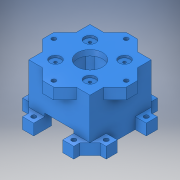
# Autodesk Inventor part: motor_holder
Saved by Autodesk Inventor 2019 (Build 230136000, 136)
## iProperties
Created: 2019-12-22
Part Number: motor_holder
Material: Пластик АБС
Document SubType Name: Modeling
Designer: Петров Иван
Density: 1.06 g/cm^3
Appearance: Голубой
Author: Петров Иван
Autodesk Inventor part; units mm, degrees
ref_plane "YZ Plane" through (0, 0, 0) normal (1, 0, 0) x (0, 1, 0)
ref_plane "XZ Plane" through (0, 0, 0) normal (0, 1, 0) x (-1, 0, 0)
ref_plane "XY Plane" through (0, 0, 0) normal (0, 0, 1) x (1, 0, 0)
sketch "Эскиз1" plane through (0, 0, 0) normal (0, 1, 0) x (-1, 0, 0)
  line L0 (-18.0075, 21.609) -> (-21.609, 18.0075)
  line L1 (-21.609, -18.0075) -> (-18.0075, -21.609)
  line L2 (18.0075, -21.609) -> (21.609, -18.0075)
  line L3 (21.609, -18.0075) -> (21.609, 18.0075)
  line L4 (21.609, 18.0075) -> (18.0075, 21.609)
  line L5 (18.0075, 21.609) -> (-18.0075, 21.609)
  circle A0 centre (0, 0) radius 11.3
  circle A1 centre (-15.5, -15.5) radius 1.25
  circle A2 centre (15.5, -15.5) radius 1.25
  circle A3 centre (15.5, 15.5) radius 1.25
  circle A4 centre (-15.5, 15.5) radius 1.25
  line L6 (13.4172, 20.8) -> (6, 20.8)
  line L7 (20.8, 13.4172) -> (13.4172, 20.8)
  line L8 (20.8, -13.4172) -> (20.8, 13.4172)
  line L9 (13.4172, -20.8) -> (20.8, -13.4172)
  line L10 (-13.4172, -20.8) -> (13.4172, -20.8)
  line L11 (-20.8, -13.4172) -> (-13.4172, -20.8)
  line L12 (-20.8, 13.4172) -> (-20.8, -13.4172)
  line L13 (-13.4172, 20.8) -> (-20.8, 13.4172)
  line L14 (-6, 20.8) -> (-13.4172, 20.8)
  line L15 (-21.609, 18.0075) -> (-21.609, -18.0075)
  line L16 (-18.0075, -21.609) -> (18.0075, -21.609)
  line L17 (-27.5, 27.5) -> (27.5, 27.5)
  line L18 (27.5, 27.5) -> (27.5, -27.5)
  line L19 (27.5, -27.5) -> (-27.5, -27.5)
  line L20 (-27.5, -27.5) -> (-27.5, 27.5)
  line L21 (-27.5, 27.5) -> (27.5, -27.5) construction
  line L22 (27.5, 27.5) -> (-27.5, -27.5) construction
  line L23 (-6, 20.8) -> (6, 20.8)
  point P0 (0, 0)
  dimension "d0" = 55
  constraints: 48 end point, 5 centre point, 2 midpoint, 2 parallel, 1 collinear, 1 horizontal, 1 perpendicular
  measures "d0" distance of L18.end L19.end
extrude "Выдавливание1" add sketch "Эскиз1" along normal blind 42 contours L17 L18 L19 L20
sketch "Эскиз3" plane through (-27.5, 0, 27.5) normal (0, 0, 1) x (1, 0, 0)
  line L0 (19.5, 0) -> (35.5, 0)
  line L1 (35.5, 0) -> (35.5, 15)
  line L2 (35.5, 15) -> (19.5, 15)
  line L3 (19.5, 15) -> (19.5, 0)
  point P0 (27.5, 0)
  dimension "d6" = 15
  constraints: 8 end point, 1 horizontal, 1 parallel, 1 perpendicular, 1 vertical
  measures "d6" distance of L1.end L0.end
extrude "Выдавливание3" cut sketch "Эскиз3" against normal blind 13.5
sketch "Эскиз4" plane through (0, 42, 0) normal (0, 1, 0) x (1, 0, 0)
  line L0 (-18.0075, 21.609) -> (-21.609, 18.0075)
  line L1 (-21.609, -18.0075) -> (-18.0075, -21.609)
  line L2 (18.0075, -21.609) -> (21.609, -18.0075)
  line L3 (21.609, -18.0075) -> (21.609, 18.0075)
  line L4 (21.609, 18.0075) -> (18.0075, 21.609)
  line L5 (18.0075, 21.609) -> (-18.0075, 21.609)
  circle A0 centre (0, 0) radius 11.3
  circle A1 centre (-15.5, -15.5) radius 1.25
  circle A2 centre (15.5, -15.5) radius 1.25
  circle A3 centre (15.5, 15.5) radius 1.25
  circle A4 centre (-15.5, 15.5) radius 1.25
  line L6 (13.4172, 20.8) -> (6, 20.8)
  line L7 (20.8, 13.4172) -> (13.4172, 20.8)
  line L8 (20.8, -13.4172) -> (20.8, 13.4172)
  line L9 (13.4172, -20.8) -> (20.8, -13.4172)
  line L10 (-13.4172, -20.8) -> (13.4172, -20.8)
  line L11 (-20.8, -13.4172) -> (-13.4172, -20.8)
  line L12 (-20.8, 13.4172) -> (-20.8, -13.4172)
  line L13 (-13.4172, 20.8) -> (-20.8, 13.4172)
  line L14 (-6, 20.8) -> (-13.4172, 20.8)
  line L15 (-21.609, 18.0075) -> (-21.609, -18.0075)
  line L16 (-18.0075, -21.609) -> (18.0075, -21.609)
  line L17 (-27.5, 27.5) -> (27.5, 27.5)
  line L18 (27.5, 27.5) -> (27.5, -27.5)
  line L19 (27.5, -27.5) -> (-27.5, -27.5)
  line L20 (-27.5, -27.5) -> (-27.5, 27.5)
  line L21 (-27.5, 27.5) -> (27.5, -27.5) construction
  line L22 (27.5, 27.5) -> (-27.5, -27.5) construction
  line L23 (-6, 20.8) -> (6, 20.8)
  point P0 (0, 0)
  dimension "d12" = 55
  constraints: 48 end point, 5 centre point, 2 midpoint, 2 parallel, 1 collinear, 1 horizontal, 1 perpendicular
  measures "d12" distance of L18.end L19.end
extrude "Выдавливание4" add sketch "Эскиз4" along normal blind 5 contours L5 L4 L3 L2 L16 L1 L15 L0 | L7 L8 L9 L10 L11 L12 L13 L14 L23 L6 | L17 L18 L19 L20
sketch "Эскиз5" plane through (0, 47, 0) normal (0, 1, 0) x (1, 0, 0)
  circle A0 centre (-15.5, -15.5) radius 1.25 projected
  circle A1 centre (-15.5, -15.5) radius 5
  circle A2 centre (-15.5, 15.5) radius 1.25 projected
  circle A3 centre (-15.5, 15.5) radius 5
  circle A4 centre (15.5, 15.5) radius 1.25 projected
  circle A5 centre (15.5, 15.5) radius 5
  circle A6 centre (15.5, -15.5) radius 1.25 projected
  circle A7 centre (15.5, -15.5) radius 5
  point P0 (0, 0)
  dimension "d15" = 10
  dimension "d16" = 10
  dimension "d17" = 10
  dimension "d18" = 10
  constraints: 4 centre point, 4 coincident
  measures "d15" diameter of A1
  measures "d16" diameter of A3
  measures "d17" diameter of A5
  measures "d18" diameter of A7
extrude "Выдавливание5" cut sketch "Эскиз5" against normal blind 2
sketch "Эскиз6" plane through (0, 0, 0) normal (0, -1, 0) x (1, 0, 0)
  line L0 (13, 27.5) -> (23, 27.5)
  line L1 (23, 27.5) -> (23, 37.5)
  line L2 (23, 37.5) -> (13, 37.5)
  line L3 (13, 37.5) -> (13, 27.5)
  line L4 (27.5, 27.5) -> (27.5, 23)
  line L5 (27.5, 23) -> (37.5, 23)
  line L6 (37.5, 23) -> (37.5, 13)
  line L7 (37.5, 13) -> (27.5, 13)
  line L8 (27.5, 13) -> (27.5, 23)
  line L9 (32.5, 23) -> (32.5, 18)
  circle A0 centre (32.5, 18) radius 2
  line L10 (23, 32.5) -> (18, 32.5)
  circle A1 centre (18, 32.5) radius 2
  line L11 (0, 0) -> (6.2032, 0)
  dimension "d22" = 10
  dimension "d23" = 10
  dimension "d24" = 4.5
  dimension "d25" = 10
  dimension "d26" = 10
  dimension "d27" = 4
  dimension "d28" = 5
  dimension "d29" = 4
  constraints: 24 end point, 4 horizontal, 4 parallel, 2 centre point, 2 coincident, 2 midpoint, 2 perpendicular, 1 vertical
  measures "d22" distance of L2.end L1.end
  measures "d23" distance of L1.end L0.end
  measures "d24" distance of L4.start L4.end
  measures "d25" distance of L6.end L7.end
  measures "d26" distance of L5.end L6.end
  measures "d27" diameter of A0
  measures "d28" distance of L10.start L10.end
  measures "d29" diameter of A1
extrude "Выдавливание6" add sketch "Эскиз6" against normal blind 10
chamfer "Фаска1" distance 4.5 angle 45 2 edges at (27.5, 5, 23) (23, 5, 27.5)
pattern_circular "Круговой массив1" count 4 over 360 about axis through (0, 42, 0) along (0, 1, 0)
sketch "Эскиз7" plane through (0, 0, 0) normal (0, -1, 0) x (1, 0, 0)
  circle A0 centre (-32.5, -18) radius 2 projected
  circle A1 centre (-18, -32.5) radius 2 projected
  line L0 (13, 27.5) -> (-13, 27.5) projected
  line L1 (-13, 27.5) -> (-13, 37.5) projected
  line L2 (-13, 37.5) -> (-23, 37.5) projected
  line L3 (-23, 37.5) -> (-23, 32) projected
  line L4 (-32, 23) -> (-23, 32) projected
  line L5 (-32, 23) -> (-37.5, 23) projected
  line L6 (-37.5, 23) -> (-37.5, 13) projected
  line L7 (-37.5, 13) -> (-27.5, 13) projected
  line L8 (-27.5, 13) -> (-27.5, -13) projected
  line L9 (-27.5, -13) -> (-37.5, -13) projected
  line L10 (-37.5, -13) -> (-37.5, -23) projected
  line L11 (-37.5, -23) -> (-32, -23) projected
  line L12 (-23, -32) -> (-32, -23) projected
  line L13 (-23, -32) -> (-23, -37.5) projected
  line L14 (-23, -37.5) -> (-13, -37.5) projected
  line L15 (-13, -37.5) -> (-13, -27.5) projected
  line L16 (-13, -27.5) -> (13, -27.5) projected
  line L17 (13, -27.5) -> (13, -37.5) projected
  line L18 (13, -37.5) -> (23, -37.5) projected
  line L19 (23, -37.5) -> (23, -32) projected
  line L20 (32, -23) -> (23, -32) projected
  line L21 (32, -23) -> (37.5, -23) projected
  line L22 (37.5, -23) -> (37.5, -13) projected
  line L23 (37.5, -13) -> (27.5, -13) projected
  line L24 (27.5, -13) -> (27.5, 13) projected
  line L25 (27.5, 13) -> (37.5, 13) projected
  line L26 (37.5, 13) -> (37.5, 23) projected
  line L27 (37.5, 23) -> (32, 23) projected
  line L28 (23, 32) -> (32, 23) projected
  line L29 (23, 32) -> (23, 37.5) projected
  line L30 (23, 37.5) -> (13, 37.5) projected
  line L31 (13, 37.5) -> (13, 27.5) projected
  circle A2 centre (-18, 32.5) radius 2 projected
  circle A3 centre (-32.5, 18) radius 2 projected
  circle A4 centre (18, -32.5) radius 2 projected
  circle A5 centre (32.5, -18) radius 2 projected
  circle A6 centre (18, 32.5) radius 2 projected
  line L32 (-18.0075, 21.609) -> (18.0075, 21.609) projected
  line L33 (18.0075, 21.609) -> (21.609, 18.0075) projected
  line L34 (21.609, 18.0075) -> (21.609, -18.0075) projected
  line L35 (21.609, -18.0075) -> (18.0075, -21.609) projected
  line L36 (18.0075, -21.609) -> (-18.0075, -21.609) projected
  line L37 (-18.0075, -21.609) -> (-21.609, -18.0075) projected
  line L38 (-21.609, -18.0075) -> (-21.609, 18.0075) projected
  line L39 (-21.609, 18.0075) -> (-18.0075, 21.609) projected
  circle A7 centre (32.5, 18) radius 2 projected
  arc A8 (0, -11.3) -> (11.3, 0) centre (0, 0) ccw projected
  arc A9 (0, -11.3) -> (11.3, 0) centre (0, 0) ccw projected
  arc A10 (0, -11.3) -> (11.3, 0) centre (0, 0) ccw projected
  arc A11 (0, -11.3) -> (11.3, 0) centre (0, 0) ccw projected
  point P0 (-11.3, 0)
  point P1 (0, 11.3)
sketch "Эскиз9" plane through (0, 47, 0) normal (0, 1, 0) x (1, 0, 0)
  line L0 (27.5, 13) -> (27.5, -13) projected
  line L1 (27.5, 0) -> (32.5, 0)
  line L2 (37.5, 5) -> (27.5, 5)
  line L3 (27.5, 5) -> (27.5, -5)
  line L4 (27.5, -5) -> (37.5, -5)
  line L5 (37.5, -5) -> (37.5, 5)
  line L6 (37.5, 5) -> (27.5, -5) construction
  line L7 (27.5, 5) -> (37.5, -5) construction
  circle A0 centre (32.5, 0) radius 1.9
  point P0 (0, 0)
  dimension "d40" = 5
  dimension "d41" = 10
  dimension "d42" = 10
  dimension "d43" = 3.8
  constraints: 14 end point, 3 midpoint, 2 horizontal, 2 parallel, 1 centre point, 1 coincident, 1 perpendicular
  measures "d40" distance of L1.start L1.end
  measures "d41" distance of L4.end L3.end
  measures "d42" distance of L3.end L2.end
  measures "d43" diameter of A0
extrude "Выдавливание8" add sketch "Эскиз9" against normal blind 10
pattern_circular "Круговой массив3" count 4 over 360 about axis through (0, 42, 0) along (0, 1, 0) of "Выдавливание8"
chamfer "Фаска4" distance 10 angle 45 8 edges at (5, 42, 27.5) (-5, 42, 27.5) (27.5, 42, 5) (27.5, 42, -5) (5, 42, -27.5) (-5, 42, -27.5) (-27.5, 42, -5) (-27.5, 42, 5)
sketch "Эскиз10" plane through (0, 47, 0) normal (0, 1, 0) x (1, 0, 0)
  line L0 (15, -27.5) -> (5, -37.5) projected
  line L1 (5, -37.5) -> (-5, -37.5) projected
  line L2 (-5, -37.5) -> (-15, -27.5) projected
  line L3 (-15, -27.5) -> (-27.5, -27.5) projected
  line L4 (-27.5, -27.5) -> (-27.5, -15) projected
  line L5 (-27.5, -15) -> (-37.5, -5) projected
  line L6 (-37.5, -5) -> (-37.5, 5) projected
  line L7 (-37.5, 5) -> (-27.5, 15) projected
  line L8 (-27.5, 15) -> (-27.5, 27.5) projected
  line L9 (-27.5, 27.5) -> (-15, 27.5) projected
  line L10 (-15, 27.5) -> (-5, 37.5) projected
  line L11 (-5, 37.5) -> (5, 37.5) projected
  line L12 (5, 37.5) -> (15, 27.5) projected
  line L13 (15, 27.5) -> (27.5, 27.5) projected
  line L14 (27.5, 27.5) -> (27.5, 15) projected
  line L15 (27.5, 15) -> (37.5, 5) projected
  line L16 (37.5, 5) -> (37.5, -5) projected
  line L17 (37.5, -5) -> (27.5, -15) projected
  line L18 (27.5, -15) -> (27.5, -27.5) projected
  line L19 (27.5, -27.5) -> (15, -27.5) projected
  circle A0 centre (0, -32.5) radius 1.9 projected
  circle A1 centre (-32.5, 0) radius 1.9 projected
  circle A2 centre (0, 32.5) radius 1.9 projected
  circle A3 centre (32.5, 0) radius 1.9 projected
  arc A4 (20.5, 15.5) -> (15.5, 20.5) centre (15.5, 15.5) ccw projected
  arc A5 (15.5, 20.5) -> (10.5, 15.5) centre (15.5, 15.5) ccw projected
  arc A6 (10.5, 15.5) -> (15.5, 10.5) centre (15.5, 15.5) ccw projected
  arc A7 (15.5, 10.5) -> (20.5, 15.5) centre (15.5, 15.5) ccw projected
  arc A8 (-10.5, -15.5) -> (-15.5, -10.5) centre (-15.5, -15.5) ccw projected
  arc A9 (-15.5, -10.5) -> (-20.5, -15.5) centre (-15.5, -15.5) ccw projected
  arc A10 (-20.5, -15.5) -> (-15.5, -20.5) centre (-15.5, -15.5) ccw projected
  arc A11 (-15.5, -20.5) -> (-10.5, -15.5) centre (-15.5, -15.5) ccw projected
  arc A12 (-10.5, 15.5) -> (-15.5, 20.5) centre (-15.5, 15.5) ccw projected
  arc A13 (-15.5, 20.5) -> (-20.5, 15.5) centre (-15.5, 15.5) ccw projected
  arc A14 (-20.5, 15.5) -> (-15.5, 10.5) centre (-15.5, 15.5) ccw projected
  arc A15 (-15.5, 10.5) -> (-10.5, 15.5) centre (-15.5, 15.5) ccw projected
  arc A16 (20.5, -15.5) -> (15.5, -10.5) centre (15.5, -15.5) ccw projected
  arc A17 (15.5, -10.5) -> (10.5, -15.5) centre (15.5, -15.5) ccw projected
  arc A18 (10.5, -15.5) -> (15.5, -20.5) centre (15.5, -15.5) ccw projected
  arc A19 (15.5, -20.5) -> (20.5, -15.5) centre (15.5, -15.5) ccw projected
  arc A20 (11.3, 0) -> (0, 11.3) centre (0, 0) ccw projected
  arc A21 (0, 11.3) -> (-11.3, 0) centre (0, 0) ccw projected
  arc A22 (-11.3, 0) -> (0, -11.3) centre (0, 0) ccw projected
  arc A23 (0, -11.3) -> (11.3, 0) centre (0, 0) ccw projected
sketch "Эскиз11" plane through (13, 0, 27.5) normal (0, 0, 1) x (1, 0, 0)
  line L0 (-26, -12.764) -> (0, -12.764)
  line L1 (0, -12.764) -> (0, 12.764)
  line L2 (0, 12.764) -> (-26, 12.764)
  line L3 (-26, 12.764) -> (-26, -12.764)
  line L4 (-26, -12.764) -> (0, 12.764) construction
  line L5 (0, -12.764) -> (-26, 12.764) construction
  line L6 (-26, 0) -> (-26, 10) projected
  point P0 (-13, 0)
  dimension "d63" = 0
  constraints: 12 end point, 2 midpoint, 2 parallel, 1 horizontal, 1 perpendicular
  measures "d63" distance between parallel lines of L6 L3
extrude "Выдавливание9" cut sketch "Эскиз11" against normal blind 10
